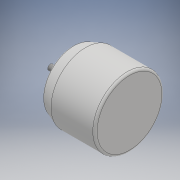
# Autodesk Inventor part: moteur
Saved by Autodesk Inventor 2018.1 (Build 221171000, 171)
## iProperties
Created: 2022-06-30
Part Number: moteur
Material: Generic
Document SubType Name: Modeling
Designer: mouta
Density: 1 g/cm^3
Appearance: Default
Author: mouta
Autodesk Inventor part; units mm, degrees
ref_plane "YZ Plane" through (0, 0, 0) normal (1, 0, 0) x (0, 1, 0)
ref_plane "XZ Plane" through (0, 0, 0) normal (0, 1, 0) x (-1, 0, 0)
ref_plane "XY Plane" through (0, 0, 0) normal (0, 0, 1) x (1, 0, 0)
sketch "Sketch1" plane through (0, 0, 0) normal (0, 0, 1) x (1, 0, 0)
  line L0 (0, 0) -> (0, 27)
  line L1 (0, 0) -> (52, 0)
  line L2 (52, 0) -> (52, 31.5)
  line L3 (52, 31.5) -> (12, 31.5)
  line L4 (12, 31.5) -> (0, 27)
  dimension "d1" = 27
  dimension "d2" = 52
  dimension "d3" = 31.5
  dimension "d4" = 40
  constraints: 10 end point, 2 perpendicular, 1 horizontal, 1 vertical
  measures "d1" distance of L0.start L0.end
  measures "d2" distance of L0.start L1.end
  measures "d3" distance of L1.end L2.end
  measures "d4" distance of L2.end L3.end
revolve "Revolution1" add sketch "Sketch1" angle 360 about axis through (0, 0, 0) along (1, 0, 0)
sketch "Sketch2" plane through (0, 0, 0) normal (-1, 0, 0) x (0, 0, 1)
  circle A0 centre (0, 0) radius 5
  dimension "d6" = 10
  constraints: 1 centre point, 1 coincident
  measures "d6" diameter of A0
extrude "Extrusion1" add sketch "Sketch2" along normal blind 2
sketch "Sketch3" plane through (-2, 0, 0) normal (-1, 0, 0) x (0, 0, 1)
  circle A0 centre (0, 0) radius 4
  dimension "d9" = 8
  constraints: 1 centre point, 1 coincident
  measures "d9" diameter of A0
extrude "Extrusion2" add sketch "Sketch3" along normal blind 12
sketch "Sketch4" plane through (-14, 0, 0) normal (-1, 0, 0) x (0, 0, 1)
  circle A0 centre (0, 0) radius 4 projected
  circle A1 centre (0, 0) radius 2.5
  dimension "d12" = 5
  constraints: 1 centre point, 1 coincident
  measures "d12" diameter of A1
extrude "Extrusion3" add sketch "Sketch4" along normal blind 6 contours A1
thread "Thread1" size "M8x1" class "6g" standard "ANSI Metric M Profile" length 6
thread "Thread2" size "M5x0.8" class "6g" standard "ANSI Metric M Profile" full length
fillet "Fillet1" radius 2 2 edges at (0, -27, 0) (52, -31.5, 0)
sketch "Sketch5" plane through (0, 0, 0) normal (-1, 0, 0) x (0, 0, 1)
  circle A0 centre (0, 15) radius 2
  circle A1 centre (0, 22) radius 2
  circle A2 centre (-15, 0) radius 2
  circle A3 centre (-22, 0) radius 2
  circle A4 centre (0, -15) radius 2
  circle A5 centre (0, -22) radius 2
  circle A6 centre (15, 0) radius 2
  circle A7 centre (22, 0) radius 2
  point P0 (0, 0)
  dimension "d20" = 4
  dimension "d21" = 4
  dimension "d24" = 360
  constraints: 8 centre point, 17 other
  measures "d20" diameter of A0
  measures "d21" diameter of A1
extrude "Extrusion4" cut sketch "Sketch5" against normal blind 8
body "Solid1"
